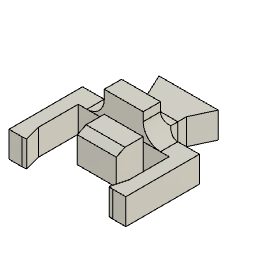
Frame-clip v24 (Autodesk Fusion 360 design; units mm, degrees)
Autodesk Fusion 360 part; units mm, degrees
sketch "Sketch1" plane through (0, 0, 0) normal (0, 0, 1) x (1, 0, 0)
  line L0 (0, 0) -> (0, 8.5)
  line L1 (13.5, 8.5) -> (13.5, 0)
  line L2 (0, 0) -> (1.5, 0)
  line L3 (1.5, 0) -> (1.5, 6.5)
  line L4 (12, 6.5) -> (12, 0)
  line L5 (12, 0) -> (13.5, 0)
  line L6 (1.5, 6.5) -> (4.5, 6.5)
  line L7 (4.5, 6.5) -> (4.5, 3.4)
  line L8 (4.5, 3.4) -> (9, 3.4)
  line L9 (9, 3.4) -> (9, 6.5)
  line L10 (9, 6.5) -> (12, 6.5)
  line L11 (4.5, 3.4) -> (9, 3.4)
  line L12 (0, 8.5) -> (4.5, 8.5)
  line L13 (4.5, 8.5) -> (4.5, 11.5)
  line L14 (4.5, 11.5) -> (3.3342, 14)
  line L15 (3.3342, 14) -> (10.1658, 14)
  line L16 (10.1658, 14) -> (9, 11.5)
  line L17 (9, 11.5) -> (9, 8.5058)
  line L18 (9, 8.5058) -> (13.5, 8.5)
  dimension "d4" = 13.5
  dimension "d5" = 1.5
  dimension "d6" = 1.5
  dimension "d8" = 3
  dimension "d9" = 3
  dimension "d11" = 3.1
  dimension "d23" = 6.5
  dimension "d31" = 3
  dimension "d32" = 155
  dimension "d34" = 155
  dimension "d36" = 2.5
  dimension "d37" = 2.5
  dimension "d49" = 2
  constraint coincident L0.start L2.start
  constraint vertical L0
  constraint horizontal L0.end L1.start
  constraint horizontal L0.start L1.end
  constraint perpendicular L0 L2
  constraint perpendicular L2 L3
  constraint perpendicular L1 L5
  constraint perpendicular L3 L6
  constraint perpendicular L6 L7
  constraint perpendicular L3 L8
  constraint perpendicular L8 L9
  constraint perpendicular L4 L10
  constraint collinear L6 L10
  constraint horizontal L11
  constraint perpendicular L7 L12
  constraint perpendicular L6 L13
  constraint horizontal L15
  constraint parallel L13 L17
  constraint collinear L7 L13
  constraint collinear L9 L17
  constraint vertical L1
  measures "d4" distance of L0.end L1.start
  measures "d5" distance of L0.start L2.end
  measures "d6" distance of L1.end L4.end
  measures "d8" distance of L3.end L6.end
  measures "d9" distance of L4.start L9.end
  measures "d11" distance of L6 L8
  measures "d23" distance of L2.end L3.end
  measures "d31" distance of L12.end L13.end
  measures "d32" angle of L13 L14
  measures "d34" angle of L16 L17
  measures "d36" distance of L13.end L15
  measures "d37" distance of L15 L16.end
  measures "d49" distance of L6 L12
extrude "Extrude2" add sketch "Sketch1" along normal blind 3
sketch "Sketch6" plane through (1.5, 0, 0) normal (1, 0, 0) x (0, 1, 0)
  line L0 (0, 0) -> (6.5, 0)
  line L1 (6.5, 0) -> (6.5, 3)
  line L2 (6.5, 3) -> (0, 3)
  line L3 (0, 3) -> (0, 0)
  line L4 (0, 0) -> (1.9, 0)
  line L5 (1.9, 0) -> (1.9, 3)
  line L6 (1.9, 3) -> (0, 3)
  line L7 (0, 3) -> (0, 0)
  dimension "d39" = 1.9
  constraint horizontal L4
  constraint vertical L5
  constraint horizontal L6
  constraint vertical L7
  constraint coincident L0.start L3.end
  measures "d39" distance of L0.start L4.end
revolve "Revolve3" add sketch "Sketch6" angle 15 about axis through (1.5, 1.9, 0) along (0, 0, 1) contours L0 L2 L3 L4 L5 L6 L7
sketch "Sketch7" plane through (12, 0, 0) normal (-1, 0, 0) x (0, -1, 0)
  line L0 (-6.5, 0) -> (0, 0)
  line L1 (0, 0) -> (0, 3)
  line L2 (0, 3) -> (-6.5, 3)
  line L3 (-6.5, 3) -> (-6.5, 0)
  line L4 (0, 3) -> (-1.9, 3)
  line L5 (-1.9, 3) -> (-1.9, 0)
  line L6 (-1.9, 0) -> (0, 0)
  line L7 (0, 0) -> (0, 3)
  dimension "d41" = 1.9
  constraint horizontal L4
  constraint vertical L5
  constraint horizontal L6
  constraint vertical L7
  constraint coincident L1.end L2.start
  measures "d41" distance of L1.end L4.end
revolve "Revolve4" add sketch "Sketch7" angle 15 about axis through (12, 1.9, 3) along (0, 0, -1) contours L0 L1 L2 L4 L5 L6 L7
sketch "Sketch8" plane through (0, 0, 3) normal (0, 0, 1) x (-1, 0, 0)
  line L0 (0, 0) -> (-1.5, 0)
  arc A0 (-1.5, 0) -> (-1.9918, -0.0647) centre (-1.5, -1.9) ccw
  line L1 (-1.9918, -0.0647) -> (-1.5, -1.9)
  line L2 (-1.5, -1.9) -> (-1.5, -6.5)
  line L3 (-1.5, -6.5) -> (-4.5, -6.5)
  line L4 (-4.5, -6.5) -> (-4.5, -3.4)
  line L5 (-4.5, -3.4) -> (-9, -3.4)
  line L6 (-9, -3.4) -> (-9, -6.5)
  line L7 (-9, -6.5) -> (-12, -6.5)
  line L8 (-12, -6.5) -> (-12, -1.9)
  line L9 (-12, -1.9) -> (-11.5082, -0.0647)
  arc A1 (-11.5082, -0.0647) -> (-12, 0) centre (-12, -1.9) ccw
  line L10 (-12, 0) -> (-13.5, 0)
  line L11 (-13.5, 0) -> (-13.5, -8.5)
  line L12 (-13.5, -8.5) -> (-9, -8.5058)
  line L13 (-9, -8.5058) -> (-9, -11.5)
  line L14 (-9, -11.5) -> (-10.1658, -14)
  line L15 (-10.1658, -14) -> (-3.3342, -14)
  line L16 (-3.3342, -14) -> (-4.5, -11.5)
  line L17 (-4.5, -11.5) -> (-4.5, -8.5)
  line L18 (-4.5, -8.5) -> (0, -8.5)
  line L19 (0, -8.5) -> (0, 0)
  line L20 (-4.5, -3.4) -> (-9, -3.4)
  line L21 (-9, -3.4) -> (-9, -8.5058)
  line L22 (-9, -8.5058) -> (-4.5, -8.5058)
  line L23 (-4.5, -8.5058) -> (-4.5, -3.4)
  constraint horizontal L20
  constraint vertical L21
  constraint horizontal L22
  constraint vertical L23
  constraint coincident L12.end L13.start
  constraint coincident L4.end L5.start
extrude "Extrude5" add sketch "Sketch8" along normal blind 0.5 contours L4 L5 L6 L17 L20 L21 L22 L23
fillet "Fillet2" radius 2 2 edges at (4.5, 8.5, 1.5) (9, 8.5058, 1.5)
chamfer "Chamfer2" distance 1 distance2 0.5 1 edges at (6.75, 3.4, 3.5) measured on face at (7.5, 6.8039, 3.5)
sketch "Sketch10" plane through (0, 0, 3.5) normal (0, 0, 1) x (-1, 0, 0)
  line L0 (-4.5, -4.4) -> (-9, -4.4)
  line L1 (-9, -4.4) -> (-9, -8.5058)
  line L2 (-9, -8.5058) -> (-4.5, -8.5058)
  line L3 (-4.5, -8.5058) -> (-4.5, -4.4)
  line L4 (-4.5, -8.5058) -> (-9, -8.5058)
  line L5 (-9, -8.5058) -> (-9, -6.5058)
  line L6 (-9, -6.5058) -> (-4.5, -6.5058)
  line L7 (-4.5, -6.5058) -> (-4.5, -8.5058)
  dimension "d52" = 2
  constraint horizontal L4
  constraint vertical L5
  constraint horizontal L6
  constraint vertical L7
  constraint coincident L2.end L3.start
  measures "d52" distance of L2.end L6.end
extrude "Extrude7" add sketch "Sketch10" along normal blind 2.5 contours L1 L2 L3 L4 L5 L6 L7
fillet "Fillet3" radius 2 3 edges at (4.5, 7.5029, 3) (6.75, 8.5058, 3) (9, 7.5029, 3)
equation "d4 = 10.4 mm + d5 + d6 + 0.1 mm"
equation "d6 = d5"
equation "d9 = d8"
equation "d11 = 4.6 mm - 1.5 mm"
equation "d32 = 155 °"
equation "d34 = d32"
equation "d37 = d36"
